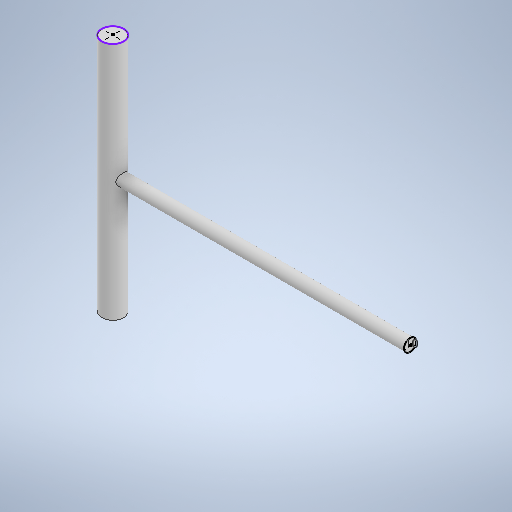
# Autodesk Inventor part: Tonbo
Saved by Autodesk Inventor 2025.1 (Build 291241000, 241)
## iProperties
Created: 2024-11-09
Part Number: Tonbo
Material: 一般
Document SubType Name: Modeling
Designer: dell
Density: 1 g/cm^3
Appearance: 既定
Author: dell
Autodesk Inventor part; units mm, degrees
ref_plane "YZ Plane" through (0, 0, 0) normal (1, 0, 0) x (0, 1, 0)
ref_plane "XZ Plane" through (0, 0, 0) normal (0, 1, 0) x (-1, 0, 0)
ref_plane "XY Plane" through (0, 0, 0) normal (0, 0, 1) x (1, 0, 0)
sketch "スケッチ1" plane through (0, 0, 0) normal (0, 1, 0) x (-1, 0, 0)
  circle A0 centre (0, 0) radius 9
  dimension "d0" = 18
  constraints: 1 centre point, 1 coincident
  measures "d0" diameter of A0
extrude "押し出し1" add sketch "スケッチ1" along normal blind 99 and the other way blind 99
sketch "スケッチ2" plane through (0, 99, 0) normal (0, 1, 0) x (1, 0, 0)
  point P0 (0, 0)
  point P1 (0, 0)
  constraints: 1 coincident
sketch "スケッチ3" plane through (0, -99, 0) normal (0, -1, 0) x (1, 0, 0)
  point P0 (0, 0)
  point P1 (0, 0)
  constraints: 1 coincident
sketch "スケッチ4" plane through (0, 0, 0) normal (1, 0, 0) x (0, 1, 0)
  point P0 (0, 0)
sketch "スケッチ5" plane through (0, 0, 0) normal (1, 0, 0) x (0, 1, 0)
  circle A0 centre (0, 0) radius 5
  dimension "d5" = 10
  constraints: 1 centre point, 1 coincident
  measures "d5" diameter of A0
extrude "押し出し2" add sketch "スケッチ5" along normal blind 246
sketch "スケッチ6" plane through (246, 0, 0) normal (1, 0, 0) x (0, 0, -1)
  point P0 (0, 0)
sketch "スケッチ7" plane through (246, 0, 0) normal (1, 0, 0) x (0, 0, -1)
  point P0 (0, 0)
sketch "スケッチ8" plane through (246, 0, 0) normal (1, 0, 0) x (0, 0, -1)
  circle A0 centre (0, 0) radius 5
  dimension "d8" = 10
  constraints: 1 centre point, 1 coincident
  measures "d8" diameter of A0
sketch "スケッチ9" plane through (0, 99, 0) normal (0, 1, 0) x (1, 0, 0)
  circle A0 centre (0, 0) radius 9
  constraints: 1 centre point, 1 coincident
